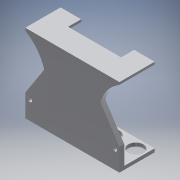
# Autodesk Inventor part: Chasis_top
Saved by Autodesk Inventor 2017 (Build 210142000, 142)
## iProperties
Created: 2018-03-01
Part Number: Chasis_top
Material: PAEK Plastic
Document SubType Name: Modeling
Designer: bradl
Density: 1.32 g/cm^3
Appearance: Smooth - White
Author: bradl
Autodesk Inventor part; units mm, degrees
ref_plane "YZ Plane" through (0, 0, 0) normal (1, 0, 0) x (0, 1, 0)
ref_plane "XZ Plane" through (0, 0, 0) normal (0, 1, 0) x (-1, 0, 0)
ref_plane "XY Plane" through (0, 0, 0) normal (0, 0, 1) x (1, 0, 0)
sketch "Sketch1" plane through (0, 0, 0) normal (0, 0, 1) x (1, 0, 0)
  line L0 (-28.0978, -20.8895) -> (-28.0978, -10.0232) projected
  line L1 (-49.931, -10.0232) -> (-28.0978, -10.0232) projected
  line L2 (-49.931, -33.6545) -> (-49.931, -10.0232) projected
  line L3 (49.9418, -33.6545) -> (-49.931, -33.6545) projected
  line L4 (49.9418, -10.0232) -> (49.9418, -33.6545) projected
  line L5 (28.0978, -10.0232) -> (49.9418, -10.0232) projected
  line L6 (28.0978, -10.0232) -> (28.0978, 46.99) projected
  line L7 (25.2422, 49.53) -> (25.2422, -14.986) projected
  line L8 (25.2422, -14.986) -> (28.0978, -14.986) projected
  line L9 (28.0978, -14.986) -> (28.0978, -20.8895) projected
  line L10 (28.0978, -20.8895) -> (-28.0978, -20.8895) projected
  line L11 (-28.0978, -16.51) -> (-28.0978, 49.53) projected
  line L12 (-28.0978, 49.53) -> (25.2422, 49.53) projected
  line L13 (49.9418, -33.6545) -> (-49.931, -33.6545)
  line L14 (-49.931, -33.6545) -> (-49.931, -30.0416)
  line L15 (-49.931, -30.0416) -> (49.9418, -30.0416)
  line L16 (49.9418, -30.0416) -> (49.9418, -33.6545)
  line L17 (49.9418, 46.99) -> (49.9418, 49.53) projected
  line L18 (28.0978, 49.53) -> (49.9418, 49.53) projected
  line L19 (28.0978, 46.99) -> (28.0978, 49.53) projected
  line L20 (28.0978, 46.99) -> (49.9418, 46.99) projected
  line L21 (-49.9418, 49.53) -> (-49.9418, 46.99) projected
  line L22 (-49.9418, 46.99) -> (-28.0978, 46.99) projected
  line L23 (-28.0978, 46.99) -> (-28.0978, 49.53) projected
  line L24 (-49.9418, 49.53) -> (-28.0978, 49.53) projected
  line L25 (49.9418, 46.99) -> (28.0978, 46.99)
  line L26 (28.0978, 46.99) -> (28.0978, 49.53)
  line L27 (28.0978, 49.53) -> (49.9418, 49.53)
  line L28 (49.9418, 49.53) -> (49.9418, 46.99)
  line L29 (-28.0978, 46.99) -> (-49.9418, 46.99)
  line L30 (-49.9418, 46.99) -> (-49.9418, 49.53)
  line L31 (-49.9418, 49.53) -> (-28.0978, 49.53)
  line L32 (-28.0978, 49.53) -> (-28.0978, 46.99)
  line L33 (28.0978, 46.99) -> (49.9418, 46.99) projected
  line L34 (49.9418, 46.99) -> (49.9418, 49.53) projected
  line L35 (49.9418, 49.53) -> (25.2422, 49.53) projected
  circle A0 centre (-44.9691, -13.9857) radius 2.286 projected
  circle A1 centre (45.2161, -14.2647) radius 2.286 projected
  point P0 (0, 0)
  constraints: 24 end point, 6 parallel, 3 horizontal, 3 perpendicular, 1 point on line
extrude "Extrusion1" add sketch "Sketch1" along normal blind 25.4 contours L22 L21 L24 L11 | L15 L4 L3 L2 | L18 L17 L20 L19
sketch "Sketch2" plane through (-49.931, -33.6545, 0) normal (0, -1, 0) x (1, 0, 0)
  circle A0 centre (9.7, 10.4) radius 8 projected
  circle A1 centre (34.9, 10.4) radius 8 projected
  circle A2 centre (64.9728, 10.4) radius 8 projected
  circle A3 centre (90.1728, 10.4) radius 8 projected
  circle A4 centre (9.7, 10.4) radius 8.128
  circle A5 centre (34.9, 10.4) radius 8.128
  circle A6 centre (64.9728, 10.4) radius 8.128
  circle A7 centre (90.1728, 10.4) radius 8.128
  point P0 (49.931, 0)
  dimension "d2" = 16.256
  dimension "d3" = 16.256
  dimension "d4" = 16.256
  dimension "d5" = 16.256
  constraints: 4 centre point, 4 coincident
  measures "d2" diameter of A4
  measures "d3" diameter of A5
  measures "d4" diameter of A6
  measures "d5" diameter of A7
extrude "Extrusion2" cut sketch "Sketch2" against normal blind 25.4 contours A0 | A1 | A2 | A3
sketch "Sketch3" plane through (0, 0, 25.4) normal (0, 0, 1) x (1, 0, 0)
  line L0 (-49.931, -33.6545) -> (49.9418, -33.6545) projected
  line L1 (49.9418, -33.6545) -> (-49.931, -33.6545)
  line L2 (-28.0978, -20.8895) -> (-28.0978, -10.0232) projected
  line L3 (-49.931, -10.0232) -> (-28.0978, -10.0232) projected
  line L4 (-49.931, -33.6545) -> (-49.931, -10.0232) projected
  line L5 (49.9418, -33.6545) -> (-49.931, -33.6545) projected
  line L6 (49.9418, -10.0232) -> (49.9418, -33.6545) projected
  line L7 (28.0978, -10.0232) -> (49.9418, -10.0232) projected
  line L8 (28.0978, -10.0232) -> (28.0978, 46.99) projected
  line L9 (28.0978, 46.99) -> (49.9418, 46.99) projected
  line L10 (49.9418, 46.99) -> (49.9418, 49.53) projected
  line L11 (49.9418, 49.53) -> (25.2422, 49.53) projected
  line L12 (25.2422, 49.53) -> (25.2422, -14.986) projected
  line L13 (25.2422, -14.986) -> (28.0978, -14.986) projected
  line L14 (28.0978, -14.986) -> (28.0978, -20.8895) projected
  line L15 (28.0978, -20.8895) -> (-28.0978, -20.8895) projected
  line L16 (-28.0978, -16.51) -> (-28.0978, 49.53) projected
  line L17 (-28.0978, 49.53) -> (25.2422, 49.53) projected
  line L18 (-28.0978, 46.99) -> (-28.0978, 49.53) projected
  line L19 (-28.0978, 49.53) -> (-49.9418, 49.53) projected
  line L20 (-49.9418, 49.53) -> (-49.9418, 46.99) projected
  line L21 (-49.9418, 46.99) -> (-28.0978, 46.99) projected
  line L22 (-49.9418, 49.53) -> (-49.9418, 46.99) projected
  line L23 (-49.9418, 46.99) -> (-49.9418, 49.53)
  line L24 (-49.9418, 49.53) -> (49.9418, 49.53)
  line L25 (49.9418, 49.53) -> (49.9418, 46.99)
  line L26 (49.9418, -30.0416) -> (-49.931, -30.0416) projected
  line L27 (-49.931, -33.6545) -> (-49.931, -30.0416)
  line L28 (49.9418, -33.6545) -> (49.9418, -30.0416)
  line L29 (49.9418, -30.0416) -> (-49.931, -30.0416) projected
  arc A0 (-49.931, -30.0416) -> (-49.9418, 46.99) centre (-72.9814, 8.471) ccw
  arc A1 (49.9418, 46.99) -> (49.9418, -30.0416) centre (72.9757, 8.4742) ccw
  point P0 (0, 0)
  constraints: 12 end point, 4 point on circle, 3 vertical, 2 centre point, 2 equal length, 2 tangent, 1 perpendicular
extrude "Extrusion3" add sketch "Sketch3" along normal blind 2.54
sketch "Sketch4" plane through (0, 0, 27.94) normal (0, 0, 1) x (1, 0, 0)
  line L0 (49.9418, -33.6545) -> (49.9418, -10.0232) projected
  line L1 (49.9418, -10.0232) -> (32.0871, -10.0232) projected
  arc A0 (49.9418, 46.99) -> (32.0871, -10.0232) centre (72.9757, 8.4742) ccw projected
  line L2 (49.9418, 46.99) -> (49.9418, 49.53) projected
  line L3 (49.9418, 49.53) -> (-49.9418, 49.53) projected
  line L4 (-49.9418, 49.53) -> (-49.9418, 46.99) projected
  arc A1 (-32.0851, -10.0232) -> (-49.9418, 46.99) centre (-72.9814, 8.471) ccw projected
  line L5 (-32.0851, -10.0232) -> (-49.931, -10.0232) projected
  line L6 (-49.931, -10.0232) -> (-49.931, -33.6545) projected
  line L7 (-49.931, -33.6545) -> (49.9418, -33.6545) projected
  line L8 (-46.121, -28.5371) -> (-46.121, -11.9877) projected
  line L9 (46.1318, -11.9877) -> (46.1318, -28.5371) projected
  line L10 (-28.0978, -16.51) -> (-28.0978, 49.53) projected
  line L11 (28.0978, -10.0232) -> (28.0978, 46.99) projected
  line L12 (-46.121, -28.5371) -> (46.1318, -28.5371)
  line L13 (46.1318, -28.5371) -> (46.1318, -11.9877)
  line L14 (46.1318, -11.9877) -> (-46.121, -11.9877)
  line L15 (-46.121, -11.9877) -> (-46.121, -28.5371)
  line L16 (-28.0978, -11.9877) -> (28.0978, -11.9877)
  line L17 (28.0978, -11.9877) -> (28.0978, -6.5147)
  line L18 (28.0978, -6.5147) -> (-28.0978, -6.5147)
  line L19 (-28.0978, -6.5147) -> (-28.0978, -11.9877)
  line L20 (-28.0978, 23.6896) -> (28.0978, 23.6896)
  line L21 (28.0978, 23.6896) -> (28.0978, 29.0198)
  line L22 (28.0978, 29.0198) -> (-28.0978, 29.0198)
  line L23 (-28.0978, 29.0198) -> (-28.0978, 23.6896)
  line L24 (-28.0978, 32.3759) -> (28.0978, 32.3759)
  line L25 (28.0978, 32.3759) -> (28.0978, 44.8129)
  line L26 (28.0978, 44.8129) -> (-28.0978, 44.8129)
  line L27 (-28.0978, 44.8129) -> (-28.0978, 32.3759)
  point P0 (0, 0)
  constraints: 32 end point, 8 parallel, 7 point on line, 4 horizontal, 4 perpendicular
extrude "Extrusion4" cut sketch "Sketch4" against normal blind 2.54 contours L11 L17 L14 L10 L18 | L20 L10 L22 L11 | L14 L9 L12 L8 | L24 L10 L26 L11
sketch "Sketch5" plane through (28.0978, 49.53, 0) normal (0, 1, 0) x (1, 0, 0)
  line L0 (0, -25.4) -> (21.844, -25.4) projected
  line L1 (-56.1955, 0) -> (-56.1955, -25.4) projected
  line L2 (0, -25.4) -> (-56.1955, -25.4)
  line L3 (-56.1955, -25.4) -> (-56.1955, -13.819)
  line L4 (-56.1955, -13.819) -> (0, -13.819)
  line L5 (0, -13.819) -> (0, -25.4)
  point P0 (-28.0978, 0)
  constraints: 8 end point, 2 parallel, 1 horizontal, 1 perpendicular, 1 point on line
extrude "Extrusion5" add sketch "Sketch5" against normal blind 2.54
sketch "Sketch6" plane through (0, 0, 27.94) normal (0, 0, 1) x (1, 0, 0)
  line L0 (46.1318, -28.5371) -> (-46.121, -28.5371) projected
  line L1 (-46.121, -11.9877) -> (-46.121, -28.5371) projected
  line L2 (28.0978, -10.0232) -> (49.9418, -10.0232) projected
  line L3 (28.0978, -11.9877) -> (46.1318, -11.9877) projected
  line L4 (28.0978, -6.5147) -> (28.0978, -11.9877) projected
  line L5 (46.1318, -28.5371) -> (46.1318, -11.9877) projected
  line L6 (46.1318, -28.5371) -> (46.1318, -11.9877) construction
  line L7 (46.1318, -11.9877) -> (28.0978, -11.9877) projected
  line L8 (46.1318, -11.9877) -> (28.0978, -11.9877) construction
  spline S0 degree 2 poles (46.1318, -28.5371) (46.1318, -11.9877) (28.0978, -11.9877) knots 1 1 1 2 2 2
  line L9 (-46.121, -28.5371) -> (-46.121, -11.9877)
  line L10 (-28.0978, -11.9877) -> (-46.121, -11.9877) projected
  line L11 (-46.121, -11.9877) -> (-28.0978, -11.9877)
  line L12 (46.1318, -28.5371) -> (46.1318, -11.9877)
  line L13 (46.1318, -11.9877) -> (28.0978, -11.9877)
  line L14 (-46.121, -11.9877) -> (-28.0978, -11.9877) projected
  line L15 (-28.0978, -11.9877) -> (-46.121, -11.9877)
  line L16 (-46.121, -11.9877) -> (-46.121, -28.5371)
  line L17 (-46.121, -28.5371) -> (-46.121, -11.9877) construction
  line L18 (-32.231, -33.6545) -> (-48.231, -33.6545) projected
  line L19 (-46.121, -11.9877) -> (-28.0978, -11.9877) construction
  spline S1 degree 2 poles (-46.121, -28.5371) (-46.121, -11.9877) (-28.0978, -11.9877) knots 1 1 1 2 2 2
  point P0 (0, 0)
  constraints: 12 end point, 7 collinear, 5 coincident, 2 perpendicular, 1 horizontal, 6 other
extrude "Extrusion6" add sketch "Sketch6" against normal blind 2.54
sketch "Sketch7" plane through (0, 0, 27.94) normal (0, 0, 1) x (1, 0, 0)
  line L0 (-28.0978, -11.9877) -> (-28.0978, -6.5147) projected
  line L1 (-28.0978, -11.9877) -> (0, -6.5147)
  line L2 (0, -6.5147) -> (28.0978, -11.9877)
  line L3 (28.0978, -11.9877) -> (28.0978, -6.5147)
  line L4 (-28.0978, -6.5147) -> (28.0978, -6.5147) projected
  line L5 (28.0978, -6.5147) -> (-28.0978, -6.5147)
  line L6 (-28.0978, -6.5147) -> (-28.0978, -11.9877)
  line L7 (0, -6.5147) -> (28.0978, -11.9877)
  line L8 (-28.0978, -11.9877) -> (-46.121, -11.9877) projected
  line L9 (-28.0978, -11.9877) -> (0, -6.5147)
  line L10 (-28.0978, -11.9877) -> (0, -6.5147)
  line L11 (0, -6.5147) -> (-28.0978, -6.5147)
  line L12 (-28.0978, -6.5147) -> (-28.0978, -11.9877)
  line L13 (0, -6.5147) -> (28.0978, -6.5147)
  line L14 (28.0978, -6.5147) -> (28.0978, -11.9877)
  line L15 (28.0978, -11.9877) -> (0, -6.5147)
  point P0 (0, 0)
  constraints: 26 end point, 4 collinear, 2 vertical, 1 perpendicular
extrude "Extrusion7" add sketch "Sketch7" against normal blind 2.54
sketch "Sketch8" plane through (0, 0, 27.94) normal (0, 0, 1) x (1, 0, 0)
  line L0 (-32.0851, -10.0232) -> (-49.931, -10.0232) projected
  line L1 (28.0978, 23.6896) -> (-28.0978, 23.6896) projected
  line L2 (-49.931, -10.0232) -> (-28.0978, 23.6896)
  line L3 (-28.0978, 23.6896) -> (28.0978, 23.6896)
  line L4 (49.9418, -10.0232) -> (32.0871, -10.0232) projected
  line L5 (28.0978, 23.6896) -> (49.9418, -10.0232)
  line L6 (49.9418, -10.0232) -> (32.0871, -10.0232)
  line L7 (0, -6.5147) -> (-28.0978, -11.9877) projected
  line L8 (32.0871, -10.0232) -> (0, -6.5147)
  line L9 (28.0978, 44.8129) -> (28.0978, 32.3759) projected
  line L10 (28.0978, 32.3759) -> (-28.0978, 32.3759) projected
  line L11 (-28.0978, 32.3759) -> (-28.0978, 44.8129) projected
  line L12 (-28.0978, 44.8129) -> (28.0978, 44.8129) projected
  line L13 (28.0978, 29.0198) -> (28.0978, 23.6896) projected
  line L14 (28.0978, 23.6896) -> (-28.0978, 23.6896) projected
  line L15 (-28.0978, 23.6896) -> (-28.0978, 29.0198) projected
  line L16 (-28.0978, 29.0198) -> (28.0978, 29.0198) projected
  line L17 (46.1318, -28.5371) -> (-46.121, -28.5371) projected
  line L18 (-28.0978, -11.9877) -> (0, -6.5147) projected
  line L19 (0, -6.5147) -> (28.0978, -11.9877) projected
  line L20 (49.9418, -33.6545) -> (49.9418, -10.0232) projected
  line L21 (49.9418, -10.0232) -> (32.0871, -10.0232) projected
  arc A0 (49.9418, 46.99) -> (32.0871, -10.0232) centre (72.9757, 8.4742) ccw projected
  line L22 (49.9418, 46.99) -> (49.9418, 49.53) projected
  line L23 (49.9418, 49.53) -> (-49.9418, 49.53) projected
  line L24 (-49.9418, 49.53) -> (-49.9418, 46.99) projected
  arc A1 (-32.0851, -10.0232) -> (-49.9418, 46.99) centre (-72.9814, 8.471) ccw projected
  line L25 (-32.0851, -10.0232) -> (-49.931, -10.0232) projected
  line L26 (-49.931, -10.0232) -> (-49.931, -33.6545) projected
  line L27 (-49.931, -33.6545) -> (49.9418, -33.6545) projected
  line L28 (0, -6.5147) -> (-32.0851, -10.0232)
  line L29 (-49.931, -10.0232) -> (-32.0851, -10.0232)
  line L30 (-49.931, -10.0232) -> (-28.0978, 23.6896)
  line L31 (-28.0978, 29.0198) -> (-28.0978, 23.6896) projected
  line L32 (-28.0978, 23.6896) -> (28.0978, 23.6896)
  line L33 (28.0978, 23.6896) -> (49.9418, -10.0232)
  line L34 (49.9418, -30.0416) -> (49.9418, -10.0232) projected
  line L35 (49.9418, -10.0232) -> (32.0871, -10.0232)
  line L36 (32.0871, -10.0232) -> (0, -6.5147)
  line L37 (-32.0851, -10.0232) -> (-49.931, -10.0232)
  point P0 (0, 0)
  constraints: 26 end point, 6 collinear, 1 horizontal, 2 other
extrude "Extrusion8" add sketch "Sketch8" against normal blind 2.54 contours L0 L2 A1 | A1 L2 L1 L5 A0 L8 L28 | A0 L5 L4
sketch "Sketch9" plane through (0, 0, 27.94) normal (0, 0, 1) x (1, 0, 0)
  line L0 (0, -6.5147) -> (-28.0978, -11.9877) projected
  line L1 (0, -6.5147) -> (28.0978, -11.9877) projected
  line L2 (-28.0978, -11.9877) -> (28.0978, -11.9877)
  line L3 (28.0978, -11.9877) -> (8.8321, -8.235)
  line L4 (28.0978, -11.9877) -> (0, -6.5147)
  line L5 (-28.0978, -11.9877) -> (0, -6.5147)
  point P0 (0, 0)
  constraints: 8 end point, 2 collinear, 1 horizontal, 1 point on line
extrude "Extrusion9" add sketch "Sketch9" against normal blind 2.54
sketch "Sketch10" plane through (0, 0, 27.94) normal (0, 0, 1) x (1, 0, 0)
  line L0 (28.0978, -11.9877) -> (-28.0978, -11.9877) construction
  line L1 (-46.121, -28.5371) -> (-28.0978, -11.9877) construction
  line L2 (-49.931, -10.0232) -> (-49.931, -30.0416) construction
  line L3 (-28.0978, -11.9877) -> (-49.931, -10.0232) construction
  line L4 (-49.931, -10.0232) -> (-37.1094, -20.2624) construction
  line L5 (46.1318, -28.5371) -> (30.9358, -11.9877) construction
  line L6 (29.8686, 20.9566) -> (49.9418, -10.0232) construction
  line L7 (30.9358, -11.9877) -> (49.9418, -10.0232) construction
  line L8 (-29.8688, 20.9549) -> (-49.931, -10.0232) construction
  line L9 (-49.931, -10.0232) -> (-44.9691, -13.9857) construction
  line L10 (-49.931, -10.0232) -> (-43.581, -10.0232) construction
  line L11 (49.9418, -10.0232) -> (38.5338, -20.2624) construction
  line L12 (49.9418, -10.0232) -> (45.2161, -14.2647) construction
  line L13 (49.9418, -10.0232) -> (56.2918, -10.0232) construction
  circle A0 centre (-44.9691, -13.9857) radius 2.286
  circle A1 centre (45.2161, -14.2647) radius 2.286
  point P0 (0, 0)
  dimension "d22" = 6.35
  dimension "d23" = 38.61
  dimension "d24" = 6.35
  dimension "d25" = 138.09
  dimension "d26" = 4.572
  dimension "d27" = 4.572
  constraints: 20 end point, 2 centre point, 2 coincident, 2 equal length, 2 horizontal, 2 midpoint, 1 perpendicular
  measures "d22" distance of L2.start L9.end
  measures "d23" angle of L9 L10
  measures "d24" distance of L6.end L12.end
  measures "d25" angle of L12 L13
  measures "d26" diameter of A0
  measures "d27" diameter of A1
extrude "Extrusion10" cut sketch "Sketch10" against normal blind 2.54
sketch "Sketch11" plane through (0, 0, 27.94) normal (0, 0, 1) x (1, 0, 0)
  circle A0 centre (-44.9691, -13.9857) radius 2.286 projected
  circle A1 centre (45.2161, -14.2647) radius 2.286 projected
  line L0 (46.1318, -28.5371) -> (-46.121, -28.5371) projected
  line L1 (-28.0978, -11.9877) -> (28.0978, -11.9877) projected
  line L2 (28.0978, 44.8129) -> (28.0978, 32.3759) projected
  line L3 (28.0978, 32.3759) -> (-28.0978, 32.3759) projected
  line L4 (-28.0978, 32.3759) -> (-28.0978, 44.8129) projected
  line L5 (-28.0978, 44.8129) -> (28.0978, 44.8129) projected
  line L6 (28.0978, 23.6896) -> (-28.0978, 23.6896) projected
  line L7 (-28.0978, 23.6896) -> (-28.0978, 29.0198) projected
  line L8 (-28.0978, 29.0198) -> (28.0978, 29.0198) projected
  line L9 (28.0978, 29.0198) -> (28.0978, 23.6896) projected
  arc A2 (49.9418, 46.99) -> (29.8686, 20.9566) centre (72.9757, 8.4742) ccw projected
  line L10 (49.9418, 46.99) -> (49.9418, 49.53) projected
  line L11 (49.9418, 49.53) -> (-49.9418, 49.53) projected
  line L12 (-49.9418, 49.53) -> (-49.9418, 46.99) projected
  arc A3 (-29.8688, 20.9549) -> (-49.9418, 46.99) centre (-72.9814, 8.471) ccw projected
  line L13 (-29.8688, 20.9549) -> (-49.931, -10.0232) projected
  line L14 (-49.931, -10.0232) -> (-49.931, -33.6545) projected
  line L15 (-49.931, -33.6545) -> (49.9418, -33.6545) projected
  line L16 (49.9418, -33.6545) -> (49.9418, -10.0232) projected
  line L17 (49.9418, -10.0232) -> (29.8686, 20.9566) projected
  line L18 (49.9418, -33.6545) -> (-49.931, -33.6545)
  line L19 (-49.931, -10.0232) -> (-49.931, -30.0416) projected
  line L20 (-49.931, -10.0232) -> (-29.8688, 20.9549)
  arc A4 (-29.8688, 20.9549) -> (-49.9418, 46.99) centre (-72.9814, 8.471) ccw
  line L21 (-49.9418, 46.99) -> (49.9418, 46.99) projected
  line L22 (-49.9418, 46.99) -> (-49.9418, 49.53)
  line L23 (49.9418, 49.53) -> (28.0978, 49.53) projected
  line L24 (-49.9418, 49.53) -> (49.9418, 49.53)
  line L25 (49.9418, 49.53) -> (49.9418, 46.99)
  line L26 (49.9418, -10.0232) -> (29.8686, 20.9566) projected
  arc A5 (49.9418, 46.99) -> (29.8686, 20.9566) centre (72.9757, 8.4742) ccw
  line L27 (29.8686, 20.9566) -> (49.9418, -10.0232)
  point P0 (0, 0)
  constraints: 12 end point, 4 point on circle, 2 centre point, 2 collinear, 1 concentric, 1 horizontal, 1 perpendicular, 1 vertical, 2 other
extrude "Extrusion11" add sketch "Sketch11" along normal blind 9.525 contours L2 L3 L4 L5 | L6 L7 L8 L9 | L21 L12 L11 L10 | A2 L17 L16 L15 L14 L13 A3 L21
sketch "Sketch12" plane through (0, 0, 25.4) normal (0, 0, -1) x (-1, 0, 0)
  circle A0 centre (44.9691, -13.9857) radius 2.286 projected
  circle A1 centre (-45.2161, -14.2647) radius 2.286 projected
  line L0 (46.121, -28.5371) -> (-46.1318, -28.5371) projected
  line L1 (-28.0978, -11.9877) -> (28.0978, -11.9877) projected
  line L2 (-28.0978, 32.3759) -> (-28.0978, 44.8129) projected
  line L3 (-28.0978, 44.8129) -> (28.0978, 44.8129) projected
  line L4 (28.0978, 44.8129) -> (28.0978, 32.3759) projected
  line L5 (28.0978, 32.3759) -> (-28.0978, 32.3759) projected
  line L6 (28.0978, 23.6896) -> (-28.0978, 23.6896) projected
  line L7 (-28.0978, 23.6896) -> (-28.0978, 29.0198) projected
  line L8 (-28.0978, 29.0198) -> (28.0978, 29.0198) projected
  line L9 (28.0978, 29.0198) -> (28.0978, 23.6896) projected
  arc A2 (49.9418, 46.99) -> (29.8688, 20.9549) centre (72.9814, 8.471) ccw projected
  line L10 (49.9418, 46.99) -> (-49.9418, 46.99) projected
  arc A3 (-29.8686, 20.9566) -> (-49.9418, 46.99) centre (-72.9757, 8.4742) ccw projected
  line L11 (-29.8686, 20.9566) -> (-49.9418, -10.0232) projected
  line L12 (-49.9418, -30.0416) -> (-49.9418, -10.0232) projected
  line L13 (-49.9418, -30.0416) -> (49.931, -30.0416) projected
  line L14 (49.931, -10.0232) -> (49.931, -30.0416) projected
  line L15 (49.931, -10.0232) -> (29.8688, 20.9549) projected
  line L16 (49.931, -30.0416) -> (-49.9418, -30.0416)
  line L17 (-49.9418, -30.0416) -> (-49.9418, -10.0232) projected
  line L18 (-49.9418, -10.0232) -> (-29.8686, 20.9566)
  arc A4 (-29.8686, 20.9566) -> (-49.9418, 46.99) centre (-72.9757, 8.4742) ccw projected
  line L19 (49.931, -10.0232) -> (49.931, -30.0416)
  line L20 (49.931, -10.0232) -> (49.931, -33.6545) projected
  line L21 (29.8688, 20.9549) -> (49.931, -10.0232) projected
  line L22 (49.931, -10.0232) -> (29.8688, 20.9549)
  line L23 (49.9418, 46.99) -> (-49.9418, 46.99)
  line L24 (-49.9418, -10.0232) -> (-49.9418, -30.0416)
  line L25 (-28.0978, 46.99) -> (-49.9418, 46.99) projected
  arc A5 (-29.8686, 20.9566) -> (-49.9418, 46.99) centre (-72.9757, 8.4742) ccw
  arc A6 (49.9418, 46.99) -> (29.8688, 20.9549) centre (72.9814, 8.471) ccw
  point P0 (0, 0)
  constraints: 12 end point, 5 point on circle, 4 collinear, 2 centre point, 1 concentric, 1 horizontal, 1 point on line, 2 other
extrude "Extrusion12" cut sketch "Sketch12" against normal blind 6.985 contours L2 L3 L4 L5 | L6 L7 L8 L9 | A2 L15 L14 L13 L12 L11 A3 L10
body "Solid1"
